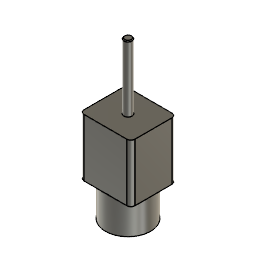
Drill Hand (Autodesk Fusion 360 design; units mm, degrees)
part number: 2026-03-29-09-31-29-809
Autodesk Fusion 360 part; units mm, degrees
sketch "Sketch1" plane through (0, 0, 0) normal (0, 0, 1) x (1, 0, 0)
  circle A0 centre (0, 0) radius 27.5
  dimension "d1" = 55
  constraint coincident A0.centre origin
  measures "d1" diameter of A0
extrude "Extrude1" add sketch "Sketch1" along normal blind 40
sketch "Sketch2" plane through (0, 0, 40) normal (0, 0, 1) x (-1, 0, 0)
  circle A0 centre (0, 0) radius 27.5
  line L0 (0, -27.5) -> (-31, -27.5)
  line L1 (-31, -27.5) -> (-31, 40.6198)
  line L2 (0, 27.5) -> (-33.618, 27.5)
  line L3 (0, -27.5) -> (31, -27.5)
  line L4 (31, -27.5) -> (31, 43)
  line L5 (0, 27.5) -> (37, 27.5)
  dimension "d4" = 90
  dimension "d5" = 31
  constraint coincident A0 L0.start
  constraint tangent A0 L0
  constraint horizontal L0
  constraint horizontal L2
  constraint coincident A0 L2.start
  constraint horizontal L3
  constraint vertical L4
  constraint perpendicular L4 L5
  measures "d4" angle of L0 L1
  measures "d5" distance of L0.start L3.end
extrude "Extrude2" add sketch "Sketch2" along normal blind 70
sketch "Sketch3" plane through (0, 0, 110) normal (0, 0, 1) x (-1, 0, 0)
  line L0 (-31, -27.5) -> (31, -27.5)
  line L1 (31, -27.5) -> (31, 27.5)
  line L2 (31, 27.5) -> (-31, 27.5)
  line L3 (-31, 27.5) -> (-31, -27.5)
  circle A0 centre (0, 0) radius 5
  dimension "d8" = 10
  constraint coincident A0.centre origin
  measures "d8" diameter of A0
extrude "Extrude3" add sketch "Sketch3" along normal blind 80 contours A0
sketch "Sketch4" plane through (0, 0, 0) normal (0, 1, 0) x (1, 0, 0)
chamfer "Chamfer1" distance 1 angle 45 1 edges at (4.6616, 1.8081, 190)
fillet "Fillet1" radius 5 4 edges at (31, -27.5, 75) (31, 27.5, 75) (-31, 27.5, 75) (-31, -27.5, 75)
